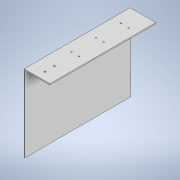
# Autodesk Inventor part: 底板3
Saved by Autodesk Inventor 2020 (Build 240168000, 168)
## iProperties
Created: 2020-12-07
Part Number: 底板3
Material: 常规
Document SubType Name: Sheet Metal
Designer: huang
Density: 1 g/cm^3
Sheet Metal Rule: 默认_mm
Appearance: 默认
Author: huang
Autodesk Inventor part; units mm, degrees
ref_plane "YZ Plane" through (0, 0, 0) normal (1, 0, 0) x (0, 1, 0)
ref_plane "XZ Plane" through (0, 0, 0) normal (0, 1, 0) x (-1, 0, 0)
ref_plane "XY Plane" through (0, 0, 0) normal (0, 0, 1) x (1, 0, 0)
sketch "草图1" plane through (0, 0, 0) normal (0, 1, 0) x (-1, 0, 0)
  line L0 (0, 0) -> (68, 0)
  line L1 (68, 0) -> (68, -280)
  line L2 (68, -280) -> (0, -280)
  line L3 (0, -280) -> (0, 0)
  line L4 (34, 0) -> (34, -21)
  circle A0 centre (34, -21) radius 2
  line L5 (34, -21) -> (34, -46)
  circle A1 centre (34, -46) radius 2
  line L6 (34, -46) -> (34, -101)
  line L7 (34, -101) -> (44, -101)
  line L8 (34, -101) -> (24, -101)
  circle A2 centre (44, -101) radius 1.5
  circle A3 centre (24, -101) radius 1.5
  line L9 (34, -101) -> (34, -166)
  line L10 (34, -166) -> (44, -166)
  line L11 (34, -166) -> (24, -166)
  circle A4 centre (44, -166) radius 1.5
  circle A5 centre (24, -166) radius 1.5
  line L12 (34, -166) -> (34, -232)
  line L13 (34, -232) -> (44, -232)
  line L14 (34, -232) -> (24, -232)
  circle A6 centre (44, -232) radius 1.5
  circle A7 centre (24, -232) radius 1.5
  dimension "d0" = 68
  dimension "d1" = 280
  dimension "d2" = 21
  dimension "d3" = 4
  dimension "d4" = 25
  dimension "d5" = 4
  dimension "d6" = 55
  dimension "d7" = 10
  dimension "d8" = 10
  dimension "d9" = 3
  dimension "d10" = 3
  dimension "d11" = 65
  dimension "d12" = 10
  dimension "d13" = 10
  dimension "d14" = 3
  dimension "d15" = 3
  dimension "d16" = 66
  dimension "d17" = 10
  dimension "d18" = 10
  dimension "d19" = 3
  dimension "d20" = 3
  constraints: 30 end point, 8 centre point, 8 coincident, 7 horizontal, 5 vertical, 2 parallel, 1 midpoint, 1 perpendicular
  measures "d0" distance of L1.end L2.end
  measures "d1" distance of L0.end L1.end
  measures "d2" distance of L4.start L4.end
  measures "d3" diameter of A0
  measures "d4" distance of L5.start L5.end
  measures "d5" diameter of A1
  measures "d6" distance of L6.start L6.end
  measures "d7" distance of L6.end L7.end
  measures "d8" distance of L6.end L8.end
  measures "d9" diameter of A2
  measures "d10" diameter of A3
  measures "d11" distance of L6.end L9.end
  measures "d12" distance of L9.end L10.end
  measures "d13" distance of L9.end L11.end
  measures "d14" diameter of A4
  measures "d15" diameter of A5
  measures "d16" distance of L9.end L12.end
  measures "d17" distance of L12.end L13.end
  measures "d18" distance of L12.end L14.end
  measures "d19" diameter of A6
  measures "d20" diameter of A7
extrude "拉伸1" add sketch "草图1" along normal blind 3
sketch "草图3" plane through (0, 0, 0) normal (0, -1, 0) x (1, 0, 0)
  line L0 (0, -280) -> (-68, -280) projected
  line L1 (-68, 0) -> (0, 0) projected
  line L2 (-68, -280) -> (-66, -280)
  line L3 (-66, -280) -> (-66, 0)
  line L4 (-66, 0) -> (-68, 0)
  line L5 (-68, 0) -> (-68, -280)
  dimension "d26" = 2
  constraints: 8 end point, 2 parallel, 1 horizontal, 1 perpendicular, 1 point on line
  measures "d26" distance between parallel lines of L5 L3
extrude "拉伸3" add sketch "草图3" along normal blind 200
equation "\"折弯半径\" = 厚度"
equation "\"折弯释压宽度\" = 厚度"
equation "\"折弯释压深度\" = 0.5 * 厚度"
equation "\"拐角释压尺寸\" = 4 * 厚度"
equation "\"最小余量\" = 2 * 厚度"
equation "\"过渡半径\" = 折弯半径"
equation "\"Jacobi半径尺寸\" = 折弯半径"
equation "\"间隙大小\" = 厚度"
equation "\"厚度\" = 0.5"
